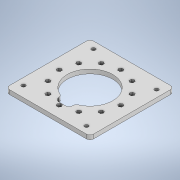
# Autodesk Inventor part: Base
Saved by Autodesk Inventor 2022 (Build 260153000, 153)
## iProperties
Created: 2022-02-26
Part Number: Base
Material: Genérico
Document SubType Name: Modeling
Designer: JK
Density: 1 g/cm^3
Appearance: Valor por defecto
Author: JK
Autodesk Inventor part; units mm, degrees
ref_plane "YZ Plane" through (0, 0, 0) normal (1, 0, 0) x (0, 1, 0)
ref_plane "XZ Plane" through (0, 0, 0) normal (0, 1, 0) x (-1, 0, 0)
ref_plane "XY Plane" through (0, 0, 0) normal (0, 0, 1) x (1, 0, 0)
sketch "Boceto1" plane through (0, 0, 0) normal (0, 1, 0) x (-1, 0, 0)
  circle A0 centre (0, 0) radius 32.5
  circle A1 centre (0, 0) radius 50.578
  dimension "d0" = 101.156
  dimension "d1" = 65
  constraints: 2 centre point, 2 coincident
  measures "d0" diameter of A1
  measures "d1" diameter of A0
extrude "Extrusión1" add sketch "Boceto1" along normal blind 6
sketch "Boceto2" plane through (0, 6, 0) normal (0, 1, 0) x (1, 0, 0)
  circle A0 centre (0, -43.944) radius 1.65
  point P0 (0, 0)
  dimension "d4" = 3.3
  dimension "d5" = 43.944
  constraints: 1 centre point
  measures "d4" diameter of A0
  measures "d5" distance of point (0, 0) A0.centre
extrude "Extrusión2" cut sketch "Boceto2" against normal through all
pattern_circular "Patrón circular1" count 12 over 360 about axis through (0, 0, 0) along (0, 1, 0) of "Extrusión2"
sketch "Boceto3" plane through (0, 0, 0) normal (0, -1, 0) x (1, 0, 0)
  line L0 (-60, -60) -> (60, -60)
  line L1 (60, -60) -> (60, 60)
  line L2 (60, 60) -> (-60, 60)
  line L3 (-60, 60) -> (-60, -60)
  line L4 (-60, -60) -> (60, 60) construction
  line L5 (60, -60) -> (-60, 60) construction
  circle A0 centre (0, 0) radius 50.578 projected
  circle A1 centre (-21.972, 38.0566) radius 1.65 projected
  circle A2 centre (-38.0566, 21.972) radius 1.65 projected
  circle A3 centre (-43.944, 0) radius 1.65 projected
  circle A4 centre (-38.0566, -21.972) radius 1.65 projected
  circle A5 centre (-21.972, -38.0566) radius 1.65 projected
  circle A6 centre (0, -43.944) radius 1.65 projected
  circle A7 centre (21.972, -38.0566) radius 1.65 projected
  circle A8 centre (38.0566, -21.972) radius 1.65 projected
  circle A9 centre (43.944, 0) radius 1.65 projected
  circle A10 centre (38.0566, 21.972) radius 1.65 projected
  circle A11 centre (21.972, 38.0566) radius 1.65 projected
  circle A12 centre (0, 43.944) radius 1.65 projected
  circle A13 centre (0, 0) radius 50.578 projected
  circle A14 centre (0, 0) radius 32.5 projected
  point P0 (0, 60)
  point P1 (60, 0)
  point P2 (0, -60)
  point P3 (-60, 0)
  dimension "d22" = 120
  dimension "d23" = 120
  constraints: 12 end point, 2 midpoint, 2 parallel, 1 horizontal, 1 perpendicular
  measures "d22" distance of L0.start L0.end
  measures "d23" distance of L0.end L1.end
extrude "Extrusión3" add sketch "Boceto3" against normal up to surface (6 mm away) contours L3 L2 L1 L0
sketch "Boceto4" plane through (0, 6, 0) normal (0, 1, 0) x (1, 0, 0)
  circle A0 centre (-45, 50) radius 2.7
  point P0 (0, 0)
  dimension "d13" = 5.4
  dimension "d14" = 45
  dimension "d16" = 50
  constraints: 1 centre point
  measures "d13" diameter of A0
  measures "d14" horizontal distance of A0.centre point (0, 0)
  measures "d16" vertical distance of A0.centre point (0, 0)
extrude "Extrusión4" cut sketch "Boceto4" against normal through all
pattern_circular "Patrón circular2" count 4 over 360 about axis through (0, 0, 0) along (0, 1, 0) of "Extrusión4"
fillet "Empalme1" radius 5 4 edges at (-60, 3, -60) (60, 3, -60) (-60, 3, 60) (60, 3, 60)
sketch "Boceto5" plane through (0, 0, 0) normal (0, -1, 0) x (1, 0, 0)
  line L0 (-10, 40) -> (10, 40)
  line L1 (10, 40) -> (10, 25)
  line L2 (10, 25) -> (-10, 25)
  line L3 (-10, 25) -> (-10, 40)
  circle A0 centre (0, 0) radius 32.5 projected
  line L4 (-10, 40) -> (10, 25) construction
  line L5 (10, 40) -> (-10, 25) construction
  point P0 (0, 32.5)
  point P1 (-10, 30.9233)
  point P2 (10, 30.9233)
  dimension "d25" = 20
  dimension "d34" = 15
  constraints: 12 end point, 2 midpoint, 2 parallel, 1 horizontal, 1 perpendicular, 2 other
  measures "d25" distance between parallel lines of L1 L3
  measures "d34" distance of L2.end L0.start
extrude "Extrusión5" cut sketch "Boceto5" against normal through all contours L0 L1 A0 L3
sketch "Boceto6" plane through (0, 6, 0) normal (0, 1, 0) x (1, 0, 0)
  circle A0 centre (-43.944, 0) radius 1.65 projected
  circle A1 centre (-43.944, 0) radius 2.85
  line L0 (-43.944, 3.2909) -> (-41.094, 1.6454)
  line L1 (-41.094, 1.6454) -> (-41.094, -1.6454)
  line L2 (-41.094, -1.6454) -> (-43.944, -3.2909)
  line L3 (-43.944, -3.2909) -> (-46.794, -1.6454)
  line L4 (-46.794, -1.6454) -> (-46.794, 1.6454)
  line L5 (-46.794, 1.6454) -> (-43.944, 3.2909)
  point P0 (0, 0)
  dimension "d28" = 5.7
  constraints: 12 end point, 2 coincident, 1 centre point, 1 tangent, 13 other
  measures "d28" diameter of A1
extrude "Extrusión6" cut sketch "Boceto6" against normal blind 4.2 contours A0 | A1 | L1 L2 A1 | A1 L0 L1 | A1 L5 L0 | L2 L3 A1 | A1 L4 L5 | L3 L4 A1
pattern_circular "Patrón circular3" count 12 over 360 about axis through (0, 0, 0) along (0, 1, 0) of "Extrusión6"
fillet "Empalme2" radius 5 4 edges at (-10, 3, 30.9233) (10, 3, 30.9233) (-10, 3, 40) (10, 3, 40)
